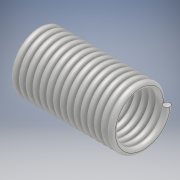
# Autodesk Inventor part: P-POD_DoorSpring
Saved by Autodesk Inventor 2018 (Build 220112000, 112)
## iProperties
Created: 2018-07-16
Part Number: P-POD_DoorSpring
Material: Stainless Steel
Document SubType Name: Modeling
Designer: Bradley
Density: 8 g/cm^3
Appearance: Semi-Polished
Author: Bradley
Autodesk Inventor part; units mm, degrees
ref_plane "YZ Plane" through (0, 0, 0) normal (1, 0, 0) x (0, 1, 0)
ref_plane "XZ Plane" through (0, 0, 0) normal (0, 1, 0) x (-1, 0, 0)
ref_plane "XY Plane" through (0, 0, 0) normal (0, 0, 1) x (1, 0, 0)
sketch "Sketch1" plane through (0, 0, 0) normal (0, 0, 1) x (1, 0, 0)
  circle A0 centre (0, 4) radius 0.5
  point P0 (0, 0)
  dimension "d0" = 1
  dimension "d1" = 4
  constraints: 1 centre point, 1 vertical alignment
  measures "d0" diameter of A0
  measures "d1" distance of point (0, 0) A0.centre
coil "Coil1" sketch "Sketch1" operation add axis through (-10, 0, 0) along (1, 0, 0) pitch 1.0667 turns 15 hand right
body "Solid1"
